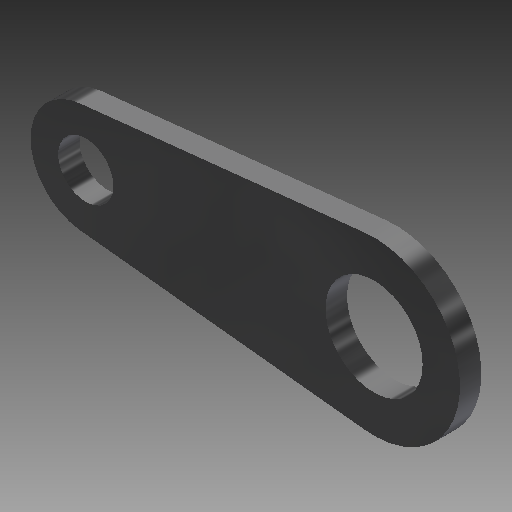
# Autodesk Inventor part: 312-01-02
Saved by Autodesk Inventor 2019 (Build 230136000, 136)
## iProperties
Company: Autodesk Inc.
Created: 2007-10-25
Part Number: 312-01-02
Document SubType Name: Modeling
Designer: Autodesk Inc.
Density: 7.85 g/cm^3
Mass: 34.6612 g
Surface Area: 33.8 cm^2
Volume: 4.41544 cm^3
Material: Steel
Description: PIVOT PLATE
Appearance: Rubber - Black - Version 1.1
Component Category: Lower Component
Author: Inventor
Autodesk Inventor part; units mm, degrees
ref_plane "YZ Plane" through (0, 0, 0) normal (1, 0, 0) x (0, 1, 0)
ref_plane "XZ Plane" through (0, 0, 0) normal (0, 1, 0) x (-1, 0, 0)
ref_plane "XY Plane" through (0, 0, 0) normal (0, 0, 1) x (1, 0, 0)
sketch "Sketch1" plane through (0, 0, 0) normal (0, 0, 1) x (1, 0, 0)
  circle A0 centre (0, 0) radius 14
  line L0 (0, 0) -> (-47, 0) construction
  circle A1 centre (-47, 0) radius 9
  line L1 (-47.9574, 8.9489) -> (-1.4894, 13.9206)
  line L2 (-47.9574, -8.9489) -> (-1.4894, -13.9206)
  dimension "d0" = 18
  dimension "d1" = 28
  dimension "d2" = 47
  constraints: 6 end point, 4 point on circle, 4 tangent, 2 centre point, 2 coincident, 1 horizontal
  measures "d0" diameter of A1
  measures "d1" diameter of A0
  measures "d2" distance of point (0, 0) L0.end
extrude "Extrusion1" add sketch "Sketch1" along normal mid plane 3.5
sketch "Sketch2" plane through (0, 0, 1.75) normal (0, 0, 1) x (1, 0, 0)
  arc A0 (-1.4894, -13.9206) -> (-1.4894, 13.9206) centre (0, 0) ccw projected
hole "Hole1" at (0, 0, 1.75) direction (0, 0, -1) diameter 15.84 end through all
sketch "Sketch3" plane through (0, 0, 1.75) normal (0, 0, 1) x (1, 0, 0)
  arc A0 (-47.9574, 8.9489) -> (-47.9574, -8.9489) centre (-47, 0) ccw projected
hole "Hole2" at (-47, 0, 1.75) direction (0, 0, -1) diameter 9 end through all
body "Solid1"
